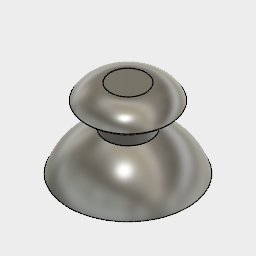
Pad_Joystick v5 (Autodesk Fusion 360 design; units mm, degrees)
Autodesk Fusion 360 part; units mm, degrees
sketch "Sketch1" plane through (0, 0, 0) normal (0, 1, 0) x (1, 0, 0)
  circle A0 centre (0, 0) radius 14.25
  dimension "d1" = 28.5
  measures "d1" diameter of A0
sphere "SpherePrimitive1" add diameter 28.5 placed x (1, 0, 0) y (0, 0, -1) z (0, 1, 0) at (0, 0, 0) makes body 1
sphere "SpherePrimitive2" cut diameter 27 placed x (1, 0, 0) y (0, 0, -1) z (0, 1, 0) at (0, 0, 0) bodies 1
box "BoxPrimitive1" cut length 30 width 30 height -15 placed x (0, 0, -1) y (-1, 0, 0) z (0, 1, 0) at (15, 0, 15) bodies 1
sketch "Sketch5" plane through (0, 0, 0) normal (0, 1, 0) x (1, 0, 0)
  circle A0 centre (0, 0) radius 5
  dimension "d9" = 10
  measures "d9" diameter of A0
extrude "Extrude1" add sketch "Sketch5" along normal blind 7 separate body makes body 2
move_body "MoveBody1" bodies 2 to x (1, 0, 0) y (0, 1, 0) z (0, 0, 1) at (0, 13, 0)
combine "Combine1" operation add target body 1 tool bodies 2
extrude "Extrude2" add 1 faces at (-0.9434, 13, -1.473) along direction (0, -1, 0) blind 6 on bodies 1 bodies 1
sketch "Sketch6" plane through (0, 7, 0) normal (0, -1, 0) x (1, 0, 0)
  circle A0 centre (0, 0) radius 3.6401
  line L0 (1.6, 2.1) -> (-1.6, 2.1)
  line L1 (-1.6, 2.1) -> (-1.6, -2.1)
  line L2 (-1.6, -2.1) -> (1.6, -2.1)
  line L3 (1.6, -2.1) -> (1.6, 2.1)
  line L4 (1.6, 2.1) -> (-1.6, -2.1) construction
  line L5 (-1.6, 2.1) -> (1.6, -2.1) construction
  dimension "d14" = 3.2
  dimension "d15" = 4.2
  constraint perpendicular L0 L1
  constraint parallel L0 L2
  constraint parallel L1 L3
  constraint horizontal L0
  constraint coincident L4
  constraint coincident L5
extrude "Extrude3" cut sketch "Sketch6" against normal blind 4.5 contours L0 L1 L2 L3 bodies 1
extrude "Extrude4" add 1 faces at (1.3101, 20, 1.9935) along direction (0, -1, 0) blind 1.656 on bodies 1 bodies 1
form "Form1" [no effect]
move_body "MoveBody2" bodies 1 to x (1, 0, 0) y (0, 1, 0) z (0, 0, 1) at (0, -4.344, 0)
box "BoxPrimitive2" cut length 30 width 30 height -6 placed x (0, 0, -1) y (-1, 0, 0) z (0, 1, 0) at (15, 0, 15) bodies 1
extrude "Extrude9" cut 1 faces at (1.3101, 15.656, 1.9935) along direction (0, -1, 0) blind 2 on bodies 1 bodies 1
extrude "Extrude10" add 1 faces at (1.3101, 13.656, 1.9935) along direction (0, 1, 0) blind 0.344 on bodies 1 bodies 1
sketch "Sketch13" plane through (0, 14, 0) normal (0, 1, 0) x (-1, 0, 0)
  circle A0 centre (0, 0) radius 5
  circle A1 centre (0, 0) radius 9.5
  dimension "d45" = 19
  constraint concentric A0 A1
  measures "d45" diameter of A1
extrude "Extrude14" add sketch "Sketch13" along normal blind 4 contours A0 | A1 bodies 1
fillet "Fillet9" radius 0.5 1 edges at (8.8571, 14, -3.4353) on bodies 1
fillet "Fillet10" radius 6 1 edges at (8.8571, 18, -3.4353) on bodies 1
fillet "Fillet11" radius 0.5 1 edges at (-4.6616, 14, 1.8081) on bodies 1
